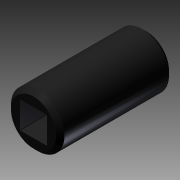
# Autodesk Inventor part: 276-1843
Saved by Autodesk Inventor 2013 (Build 170138000, 138)
## iProperties
Category: Motion
Company: Autodesk Inc.
Created: 2012-03-23
Part Number: 276-1843
Document SubType Name: Modeling
Designer: Autodesk Inc.
Density: 7.85 g/cm^3
Material: Steel
Catalog Web Link: http://www.vexrobotics.com/276-1843.html
Vendor: VEX
Mass: 2.31571 g
Surface Area: 4.72907 cm^2
Volume: 0.294995 cm^3
Author: Autodesk Inc.
Autodesk Inventor part; units mm, degrees
ref_plane "YZ Plane" through (0, 0, 0) normal (1, 0, 0) x (0, 1, 0)
ref_plane "XZ Plane" through (0, 0, 0) normal (0, 1, 0) x (-1, 0, 0)
ref_plane "XY Plane" through (0, 0, 0) normal (0, 0, 1) x (1, 0, 0)
sketch "Sketch1" plane through (0, 0, 0) normal (0, 0, 1) x (1, 0, 0)
  circle A0 centre (0, 0) radius 3.2
  dimension "d0" = 6.4
  constraints: 1 centre point, 1 coincident
  measures "d0" diameter of A0
extrude "Extrusion1" add sketch "Sketch1" against normal blind 13.5
sketch "Sketch2" plane through (0, 0, 0) normal (0, 0, 1) x (1, 0, 0)
  circle A0 centre (0, 0) radius 2.7
  line L0 (1.6129, -1.5129) -> (1.6129, 1.5129)
  arc A1 (1.5129, -1.6129) -> (1.6129, -1.5129) centre (1.5129, -1.5129) ccw
  line L1 (-1.5129, -1.6129) -> (1.5129, -1.6129)
  arc A2 (-1.6129, -1.5129) -> (-1.5129, -1.6129) centre (-1.5129, -1.5129) ccw
  line L2 (-1.6129, 1.5129) -> (-1.6129, -1.5129)
  arc A3 (-1.5129, 1.6129) -> (-1.6129, 1.5129) centre (-1.5129, 1.5129) ccw
  line L3 (1.5129, 1.6129) -> (-1.5129, 1.6129)
  arc A4 (1.6129, 1.5129) -> (1.5129, 1.6129) centre (1.5129, 1.5129) ccw
  constraints: 8 end point, 8 point on circle, 5 centre point
extrude "Extrusion2" cut sketch "Sketch2" against normal blind 5.75 contours A1 L1 A2 L2 A3 L3 A4 L0
sketch "Sketch3" plane through (0, 0, -13.5) normal (0, 0, -1) x (-1, 0, 0)
  circle A0 centre (0, 0) radius 2.7
  line L0 (1.6129, -1.5129) -> (1.6129, 1.5129)
  arc A1 (1.5129, -1.6129) -> (1.6129, -1.5129) centre (1.5129, -1.5129) ccw
  line L1 (-1.5129, -1.6129) -> (1.5129, -1.6129)
  arc A2 (-1.6129, -1.5129) -> (-1.5129, -1.6129) centre (-1.5129, -1.5129) ccw
  line L2 (-1.6129, 1.5129) -> (-1.6129, -1.5129)
  arc A3 (-1.5129, 1.6129) -> (-1.6129, 1.5129) centre (-1.5129, 1.5129) ccw
  line L3 (1.5129, 1.6129) -> (-1.5129, 1.6129)
  arc A4 (1.6129, 1.5129) -> (1.5129, 1.6129) centre (1.5129, 1.5129) ccw
  constraints: 8 end point, 8 point on circle, 5 centre point
extrude "Extrusion3" cut sketch "Sketch3" against normal blind 5.4 contours A1 L1 A2 L2 A3 L3 A4 L0
sketch "Sketch4" plane through (0, 0, -8.1) normal (0, 0, -1) x (-1, 0, 0)
  circle A0 centre (0, 0) radius 1.5875
  dimension "d7" = 3.175
  constraints: 1 centre point, 1 coincident
  measures "d7" diameter of A0
extrude "Extrusion4" cut sketch "Sketch4" against normal up to next
chamfer "Chamfer1" distance 0.5 angle 45 2 edges at (-3.2, 0, -13.5) (-3.2, 0, 0)
sketch "Sketch5" plane through (0, 0, 0) normal (0, 0, 1) x (1, 0, 0)
  line L0 (1.6129, 1.5129) -> (1.6129, -1.5129) projected
  line L1 (1.5129, -1.6129) -> (-1.5129, -1.6129) projected
  line L2 (-1.6129, -1.5129) -> (-1.6129, 1.5129) projected
  line L3 (-1.5129, 1.6129) -> (1.5129, 1.6129) projected
  circle A0 centre (0, 0) radius 2.7 projected
  circle A1 centre (0, 0) radius 1.6129
  constraints: 4 tangent, 1 centre point, 1 coincident
surface extrude "ExtrusionSrf1" sketch "Sketch5" against normal up to surface (13.5 mm away) shown no curves A1
body "Solid1"
body "Srf1"
